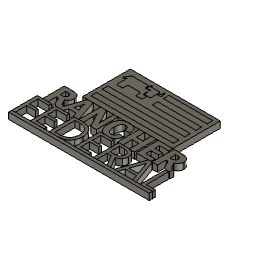
rancher-federal-stand (Autodesk Fusion 360 design; units mm, degrees)
Autodesk Fusion 360 part; units mm, degrees
sketch "Sketch1" plane through (0, 0, 0) normal (0, 0, 1) x (1, 0, 0)
  line L0 (14.2062, -89.6558) -> (3.2469, -89.6558)
  line L1 (3.2469, -89.6558) -> (-8.7202, -125.3052)
  spline S0 degree 3 poles (-8.7202, -125.3052) (-9.2241, -125.4312) (-9.791, -125.5571) (-10.2948, -125.5571) knots 0 0 0 0 1 1 1 1
  spline S1 degree 3 poles (-10.2948, -125.5571) (-14.1369, -125.5571) (-15.3336, -121.4631) (-17.1602, -117.81) knots 0 0 0 0 1 1 1 1
  spline S2 degree 3 poles (-17.1602, -117.81) (-17.853, -116.2354) (-18.9237, -114.7867) (-20.1834, -113.653) knots 0 0 0 0 1 1 1 1
  spline S3 degree 3 poles (-20.1834, -113.653) (-15.8375, -112.2673) (-11.3656, -108.3623) (-11.3656, -101.8119) knots 0 0 0 0 1 1 1 1
  spline S4 degree 3 poles (-11.3656, -101.8119) (-11.3656, -93.8128) (-17.0972, -89.6558) (-25.6631, -89.6558) knots 0 0 0 0 1 1 1 1
  line L2 (-25.6631, -89.6558) -> (-43.6138, -89.6558)
  line L3 (-43.6138, -89.6558) -> (-43.6138, -133.3683)
  line L4 (-43.6138, -133.3683) -> (-32.7804, -133.3683)
  line L5 (-32.7804, -133.3683) -> (-32.7804, -115.9834)
  line L6 (-32.7804, -115.9834) -> (-30.324, -115.9834)
  spline S5 degree 3 poles (-30.324, -115.9834) (-27.9306, -115.9834) (-26.104, -121.4631) (-24.8443, -124.5494) knots 0 0 0 0 1 1 1 1
  spline S6 degree 3 poles (-24.8443, -124.5494) (-21.821, -131.4777) (-18.8607, -133.4932) (-13.696, -133.4932) knots 0 0 0 0 1 1 1 1
  spline S7 degree 3 poles (-13.696, -133.4932) (-12.9402, -133.4302) (-12.1844, -133.3672) (-11.4285, -133.3042) knots 0 0 0 0 1 1 1 1
  line L7 (-11.4285, -133.3042) -> (-1.9808, -133.3042)
  line L8 (-1.9808, -133.3042) -> (0.6645, -124.9903)
  line L9 (0.6645, -124.9903) -> (15.277, -124.9903)
  line L10 (15.277, -124.9903) -> (18.0267, -133.4312)
  line L11 (18.0267, -133.4312) -> (28.9876, -133.4312)
  line L12 (28.9876, -133.4312) -> (14.2062, -89.6558)
  line L13 (-28.9383, -108.2363) -> (-32.8434, -108.2363)
  line L14 (-32.8434, -108.2363) -> (-32.8434, -97.5289)
  line L15 (-32.8434, -97.5289) -> (-27.6157, -97.5289)
  spline S8 degree 3 poles (-27.6157, -97.5289) (-24.6554, -97.5289) (-22.199, -98.7886) (-22.199, -102.6307) knots 0 0 0 0 1 1 1 1
  spline S9 degree 3 poles (-22.199, -102.6307) (-22.199, -107.2915) (-25.8521, -108.2363) (-28.9383, -108.2363) knots 0 0 0 0 1 1 1 1
  line L16 (3.2469, -117.0542) -> (6.2701, -107.7954)
  spline S10 degree 3 poles (6.2701, -107.7954) (7.026, -105.339) (7.5298, -102.8826) (7.9078, -100.3632) knots 0 0 0 0 1 1 1 1
  line L17 (7.9078, -100.3632) -> (8.1597, -100.3632)
  spline S11 degree 3 poles (8.1597, -100.3632) (8.4746, -102.8826) (8.9785, -105.402) (9.6713, -107.8584) knots 0 0 0 0 1 1 1 1
  line L18 (9.6713, -107.8584) -> (12.6316, -117.0542)
  line L19 (12.6316, -117.0542) -> (3.2469, -117.0542)
  line L20 (29.3856, -89.6558) -> (40.9747, -89.6558)
  line L21 (40.9747, -89.6558) -> (52.438, -111.3226)
  spline S12 degree 3 poles (52.438, -111.3226) (53.3828, -113.2121) (54.7054, -116.4873) (55.7132, -119.0697) knots 0 0 0 0 1 1 1 1
  line L22 (55.7132, -119.0697) -> (55.9651, -119.0697)
  spline S13 degree 3 poles (55.9651, -119.0697) (55.8392, -116.6133) (55.5242, -113.0861) (55.5242, -110.5668) knots 0 0 0 0 1 1 1 1
  line L23 (55.5242, -110.5668) -> (55.5242, -89.6558)
  line L24 (55.5242, -89.6558) -> (64.4051, -89.6558)
  line L25 (64.4051, -89.6558) -> (64.4051, -133.3043)
  line L26 (64.4051, -133.3043) -> (53.0678, -133.3043)
  line L27 (53.0678, -133.3043) -> (41.1637, -111.7005)
  spline S14 degree 3 poles (41.1637, -111.7005) (39.967, -109.37) (38.8963, -107.0396) (38.0145, -104.5832) knots 0 0 0 0 1 1 1 1
  line L28 (38.0145, -104.5832) -> (37.7625, -104.5832)
  spline S15 degree 3 poles (37.7625, -104.5832) (37.9515, -107.0396) (38.2664, -109.9369) (38.2664, -112.3303) knots 0 0 0 0 1 1 1 1
  line L29 (38.2664, -112.3303) -> (38.2664, -133.4313)
  line L30 (38.2664, -133.4313) -> (29.3226, -133.4313)
  line L31 (29.3226, -133.4313) -> (29.3226, -89.6558)
  line L32 (29.3226, -89.6558) -> (29.3856, -89.6558)
  spline S16 degree 3 poles (66.6725, -111.1966) (66.6725, -95.3874) (74.4826, -88.9) (86.5757, -88.9) knots 0 0 0 0 1 1 1 1
  spline S17 degree 3 poles (86.5757, -88.9) (99.2986, -88.9) (104.4634, -95.8913) (103.0147, -105.339) knots 0 0 0 0 1 1 1 1
  line L33 (103.0147, -105.339) -> (92.9372, -106.2208)
  spline S18 degree 3 poles (92.9372, -106.2208) (94.0709, -99.2925) (91.2996, -96.5212) (86.3868, -96.5212) knots 0 0 0 0 1 1 1 1
  spline S19 degree 3 poles (86.3868, -96.5212) (81.6629, -96.5212) (77.8208, -100.0483) (77.8208, -111.2596) knots 0 0 0 0 1 1 1 1
  spline S20 degree 3 poles (77.8208, -111.2596) (77.8208, -123.1637) (81.9778, -126.187) (86.7017, -126.187) knots 0 0 0 0 1 1 1 1
  spline S21 degree 3 poles (86.7017, -126.187) (91.1736, -126.187) (94.7637, -123.4156) (94.0079, -117.684) knots 0 0 0 0 1 1 1 1
  line L34 (94.0079, -117.684) -> (103.4556, -118.6288)
  spline S22 degree 3 poles (103.4556, -118.6288) (104.1484, -127.5097) (97.787, -133.9971) (86.1348, -133.9971) knots 0 0 0 0 1 1 1 1
  spline S23 degree 3 poles (86.1348, -133.9971) (74.3567, -134.1231) (66.7355, -127.1317) (66.6725, -111.1966) knots 0 0 0 0 1 1 1 1
  line L35 (106.9828, -89.6558) -> (117.7532, -89.6558)
  line L36 (117.7532, -89.6558) -> (117.7532, -106.1578)
  line L37 (117.7532, -106.1578) -> (131.0429, -106.1578)
  line L38 (131.0429, -106.1578) -> (131.0429, -89.6558)
  line L39 (131.0429, -89.6558) -> (141.8133, -89.6558)
  line L40 (141.8133, -89.6558) -> (141.8133, -134.1292)
  line L41 (141.8133, -134.1292) -> (131.0429, -134.1292)
  line L42 (131.0429, -134.1292) -> (131.0429, -114.8497)
  line L43 (131.0429, -114.8497) -> (117.7532, -114.8497)
  line L44 (117.7532, -114.8497) -> (117.7532, -133.3672)
  line L45 (117.7532, -133.3672) -> (106.9828, -133.3672)
  line L46 (106.9828, -133.3672) -> (106.9828, -89.6558)
  line L47 (144.8996, -89.6558) -> (173.8096, -89.6558)
  line L48 (173.8096, -89.6558) -> (173.8096, -97.7179)
  line L49 (173.8096, -97.7179) -> (155.733, -97.7179)
  line L50 (155.733, -97.7179) -> (155.733, -107.1026)
  line L51 (155.733, -107.1026) -> (170.9123, -107.1026)
  line L52 (170.9123, -107.1026) -> (170.9123, -115.1017)
  line L53 (170.9123, -115.1017) -> (155.733, -115.1017)
  line L54 (155.733, -115.1017) -> (155.733, -125.3052)
  line L55 (155.733, -125.3052) -> (174.4394, -125.3052)
  line L56 (174.4394, -125.3052) -> (174.4394, -133.6974)
  line L57 (174.4394, -133.6974) -> (144.8996, -133.6974)
  line L58 (144.8996, -133.6974) -> (144.8996, -89.6558)
  line L59 (176.5179, -89.6558) -> (194.4686, -89.6558)
  spline S24 degree 3 poles (194.4686, -89.6558) (203.0345, -89.6558) (208.7662, -93.8128) (208.7662, -101.8119) knots 0 0 0 0 1 1 1 1
  spline S25 degree 3 poles (208.7662, -101.8119) (208.7662, -108.3623) (204.2942, -112.2673) (199.9483, -113.653) knots 0 0 0 0 1 1 1 1
  spline S26 degree 3 poles (199.9483, -113.653) (201.208, -114.7867) (202.2787, -116.2354) (202.9715, -117.81) knots 0 0 0 0 1 1 1 1
  spline S27 degree 3 poles (202.9715, -117.81) (204.7981, -121.4631) (205.9948, -125.5571) (209.8369, -125.5571) knots 0 0 0 0 1 1 1 1
  spline S28 degree 3 poles (209.8369, -125.5571) (210.4038, -125.5571) (211.0336, -125.4312) (211.6005, -125.2422) knots 0 0 0 0 1 1 1 1
  line L60 (211.6005, -125.2422) -> (210.7817, -132.9263)
  spline S29 degree 3 poles (210.7817, -132.9263) (209.333, -133.2413) (207.8844, -133.4302) (206.4357, -133.4932) knots 0 0 0 0 1 1 1 1
  spline S30 degree 3 poles (206.4357, -133.4932) (201.2709, -133.4932) (198.3107, -131.4777) (195.2244, -124.5494) knots 0 0 0 0 1 1 1 1
  spline S31 degree 3 poles (195.2244, -124.5494) (193.9647, -121.4631) (192.1382, -115.9834) (189.7447, -115.9834) knots 0 0 0 0 1 1 1 1
  line L61 (189.7447, -115.9834) -> (187.2883, -115.9834)
  line L62 (187.2883, -115.9834) -> (187.2883, -133.7493)
  line L63 (187.2883, -133.7493) -> (176.5179, -133.7493)
  line L64 (176.5179, -133.7493) -> (176.5179, -89.6558)
  line L65 (187.3513, -97.5289) -> (187.3513, -108.2363)
  line L66 (187.3513, -108.2363) -> (191.2564, -108.2363)
  spline S32 degree 3 poles (191.2564, -108.2363) (194.3427, -108.2363) (197.9958, -107.2915) (197.9958, -102.6307) knots 0 0 0 0 1 1 1 1
  spline S33 degree 3 poles (197.9958, -102.6307) (197.9958, -98.7886) (195.5394, -97.5289) (192.5791, -97.5289) knots 0 0 0 0 1 1 1 1
  line L67 (192.5791, -97.5289) -> (187.3513, -97.5289)
  line L68 (77.6602, -0.8188) -> (165.5239, -0.8188)
  line L69 (165.5239, -0.8188) -> (165.5239, -12.0931)
  line L70 (165.5239, -12.0931) -> (77.6602, -12.0931)
  line L71 (77.6602, -12.0931) -> (77.6602, -0.8188)
  line L72 (77.6602, -23.3673) -> (165.5239, -23.3673)
  line L73 (165.5239, -23.3673) -> (165.5239, -34.6416)
  line L74 (165.5239, -34.6416) -> (77.6602, -34.6416)
  line L75 (77.6602, -34.6416) -> (77.6602, -23.3673)
  line L76 (0, -45.9159) -> (165.5239, -45.9159)
  line L77 (165.5239, -45.9159) -> (165.5239, -57.1902)
  line L78 (165.5239, -57.1902) -> (0, -57.1902)
  line L79 (0, -57.1902) -> (0, -45.9159)
  line L80 (0, -68.5274) -> (165.5239, -68.5274)
  line L81 (165.5239, -68.5274) -> (165.5239, -79.8017)
  line L82 (165.5239, -79.8017) -> (0, -79.8017)
  line L83 (0, -79.8017) -> (0, -68.5274)
  line L84 (72.0546, -8.251) -> (71.2987, -3.5901)
  spline S34 degree 3 poles (71.2987, -3.5901) (71.0468, -2.0785) (70.4799, -0.8188) (69.9761, -0.8188) knots 0 0 0 0 1 1 1 1
  spline S35 degree 3 poles (69.9761, -0.8188) (69.4722, -0.8188) (69.1573, -2.0785) (69.1573, -3.5901) knots 0 0 0 0 1 1 1 1
  line L85 (69.1573, -3.5901) -> (69.1573, -4.8498)
  spline S36 degree 3 poles (69.1573, -4.8498) (69.1573, -6.3615) (67.8976, -7.5582) (66.3859, -7.5582) knots 0 0 0 0 1 1 1 1
  line L86 (66.3859, -7.5582) -> (64.8743, -7.5582)
  line L87 (64.8743, -7.5582) -> (64.8743, -10.9593)
  line L88 (64.8743, -10.9593) -> (69.7871, -10.9593)
  spline S37 degree 3 poles (69.7871, -10.9593) (71.0468, -11.0223) (72.1175, -10.0146) (72.1805, -8.7549) knots 0 0 0 0 1 1 1 1
  spline S38 degree 3 poles (72.1805, -8.7549) (72.1175, -8.5659) (72.1175, -8.377) (72.0546, -8.251) knots 0 0 0 0 1 1 1 1
  line L89 (61.0322, -4.283) -> (45.6639, -4.283)
  spline S39 degree 3 poles (45.6639, -4.283) (45.601, -4.283) (45.475, -4.283) (45.412, -4.283) knots 0 0 0 0 1 1 1 1
  line L90 (45.412, -4.283) -> (45.412, -3.5271)
  spline S40 degree 3 poles (45.412, -3.5271) (45.412, -2.0155) (45.0341, -0.7558) (44.5932, -0.7558) knots 0 0 0 0 1 1 1 1
  spline S41 degree 3 poles (44.5932, -0.7558) (44.1523, -0.7558) (43.5225, -2.0155) (43.2705, -3.4642) knots 0 0 0 0 1 1 1 1
  line L91 (43.2705, -3.4642) -> (42.4517, -8.188)
  spline S42 degree 3 poles (42.4517, -8.188) (42.1998, -9.4477) (42.9556, -10.6444) (44.2153, -10.8964) knots 0 0 0 0 1 1 1 1
  spline S43 degree 3 poles (44.2153, -10.8964) (44.4043, -10.9593) (44.5932, -10.9593) (44.7822, -10.9593) knots 0 0 0 0 1 1 1 1
  line L92 (44.7822, -10.9593) -> (49.3801, -10.9593)
  spline S44 degree 3 poles (49.3801, -10.9593) (49.8209, -10.9593) (50.2618, -10.8964) (50.7027, -10.7074) knots 0 0 0 0 1 1 1 1
  spline S45 degree 3 poles (50.7027, -10.7074) (50.5768, -11.5262) (49.8839, -12.0931) (49.0651, -12.0931) knots 0 0 0 0 1 1 1 1
  line L93 (49.0651, -12.0931) -> (42.5777, -12.0931)
  spline S46 degree 3 poles (42.5777, -12.0931) (41.6329, -12.0931) (40.8771, -11.3373) (40.8771, -10.3925) knots 0 0 0 0 1 1 1 1
  spline S47 degree 3 poles (40.8771, -10.3925) (40.8771, -10.3295) (40.8771, -10.2035) (40.8771, -10.1405) knots 0 0 0 0 1 1 1 1
  line L94 (40.8771, -10.1405) -> (41.507, -6.2355)
  spline S48 degree 3 poles (41.507, -6.2355) (41.6329, -5.2907) (41.0661, -4.4719) (40.1213, -4.283) knots 0 0 0 0 1 1 1 1
  spline S49 degree 3 poles (40.1213, -4.283) (40.0583, -4.283) (39.9323, -4.283) (39.8693, -4.283) knots 0 0 0 0 1 1 1 1
  line L95 (39.8693, -4.283) -> (7.6841, -4.283)
  spline S50 degree 3 poles (7.6841, -4.283) (6.9913, -4.283) (6.4244, -4.6609) (6.1725, -5.2907) knots 0 0 0 0 1 1 1 1
  line L96 (6.1725, -5.2907) -> (0.063, -14.4865)
  spline S51 degree 3 poles (0.063, -14.4865) (-0.063, -14.6125) (0, -14.8644) (0.063, -14.9904) knots 0 0 0 0 1 1 1 1
  line L97 (0.063, -14.9904) -> (1.2597, -16.376)
  spline S52 degree 3 poles (1.2597, -16.376) (1.3857, -16.565) (1.6376, -16.565) (1.8266, -16.439) knots 0 0 0 0 1 1 1 1
  line L98 (1.8266, -16.439) -> (5.9206, -13.2268)
  line L99 (5.9206, -13.2268) -> (5.9206, -32.941)
  spline S53 degree 3 poles (5.9206, -32.941) (5.9206, -33.8858) (6.6764, -34.6416) (7.5582, -34.6416) knots 0 0 0 0 1 1 1 1
  line L100 (7.558, -34.6416) -> (16.7539, -34.6416)
  spline S54 degree 3 poles (16.7539, -34.6416) (17.6987, -34.6416) (18.4545, -33.8858) (18.4545, -32.941) knots 0 0 0 0 1 1 1 1
  line L101 (18.4545, -32.941) -> (18.4545, -26.0757)
  spline S55 degree 3 poles (18.4545, -26.0757) (18.4545, -25.1309) (19.2104, -24.3751) (20.1551, -24.3751) knots 0 0 0 0 1 1 1 1
  line L102 (20.1551, -24.3751) -> (42.9556, -24.3751)
  spline S56 degree 3 poles (42.9556, -24.3751) (43.9004, -24.3751) (44.6562, -25.1309) (44.6562, -26.0757) knots 0 0 0 0 1 1 1 1
  line L103 (44.6562, -26.0757) -> (44.6562, -32.941)
  spline S57 degree 3 poles (44.6562, -32.941) (44.6562, -33.8858) (45.412, -34.6416) (46.2938, -34.6416) knots 0 0 0 0 1 1 1 1
  line L104 (46.2938, -34.6416) -> (55.4896, -34.6416)
  spline S58 degree 3 poles (55.4896, -34.6416) (56.4343, -34.6416) (57.1901, -33.8858) (57.1901, -32.941) knots 0 0 0 0 1 1 1 1
  line L105 (57.1901, -32.941) -> (57.1901, -25.5088)
  line L106 (57.1901, -25.5088) -> (52.3403, -25.5088)
  spline S59 degree 3 poles (52.3403, -25.5088) (50.8287, -25.5088) (49.569, -24.2491) (49.569, -22.7375) knots 0 0 0 0 1 1 1 1
  line L107 (49.569, -22.7375) -> (49.569, -18.0136)
  spline S60 degree 3 poles (49.569, -18.0136) (49.569, -17.1319) (50.0099, -16.313) (50.7027, -15.8092) knots 0 0 0 0 1 1 1 1
  line L108 (50.7027, -15.8092) -> (50.7027, -21.4778)
  spline S61 degree 3 poles (50.7027, -21.4778) (50.7027, -22.9894) (51.9624, -24.2491) (53.4741, -24.2491) knots 0 0 0 0 1 1 1 1
  line L109 (53.4741, -24.2491) -> (60.9063, -24.2491)
  spline S62 degree 3 poles (60.9063, -24.2491) (62.4179, -24.2491) (63.6776, -22.9894) (63.6776, -21.4778) knots 0 0 0 0 1 1 1 1
  line L110 (63.6776, -21.4778) -> (63.6776, -6.9913)
  spline S63 degree 3 poles (63.6776, -6.9913) (63.7406, -5.4797) (62.5439, -4.283) (61.0322, -4.283) knots 0 0 0 0 1 1 1 1
  line L111 (-6.9304, 6.1202) -> (173.8096, 6.1202)
  line L112 (173.8096, 6.1202) -> (173.8096, -89.6558)
  line L113 (173.8096, -89.6558) -> (-6.9304, -89.6558)
  line L114 (-6.9304, -89.6558) -> (-6.9304, 6.1202)
  line L115 (-25.4398, -133.357) -> (-25.4398, -138.7816)
  line L116 (-25.4398, -138.7816) -> (-47.6511, -138.7816)
  line L117 (-47.6511, -138.7816) -> (-47.6511, -156.0081)
  line L118 (-47.6511, -156.0081) -> (-29.6182, -156.0081)
  line L119 (-29.6182, -156.0081) -> (-29.6182, -161.4326)
  line L120 (-29.6182, -161.4326) -> (-47.6511, -161.4326)
  line L121 (-47.6511, -161.4326) -> (-47.6511, -184.4502)
  line L122 (-47.6511, -184.4502) -> (-54.3218, -184.4502)
  line L123 (-54.3218, -184.4502) -> (-54.3218, -133.357)
  line L124 (-54.3218, -133.357) -> (-25.4398, -133.357)
  line L125 (-10.7056, -138.7816) -> (-10.7056, -155.8615)
  line L126 (-10.7056, -155.8615) -> (7.9137, -155.8615)
  line L127 (7.9137, -155.8615) -> (7.9137, -161.3593)
  line L128 (7.9137, -161.3593) -> (-10.7056, -161.3593)
  line L129 (-10.7056, -161.3593) -> (-10.7056, -178.9524)
  line L130 (-10.7056, -178.9524) -> (10.1128, -178.9524)
  line L131 (10.1128, -178.9524) -> (10.1128, -184.4502)
  line L132 (10.1128, -184.4502) -> (-17.3763, -184.4502)
  line L133 (-17.3763, -184.4502) -> (-17.3763, -133.2837)
  line L134 (-17.3763, -133.2837) -> (10.1128, -133.2837)
  line L135 (10.1128, -133.2837) -> (10.1128, -138.7816)
  line L136 (10.1128, -138.7816) -> (-10.7056, -138.7816)
  spline S64 degree 2 poles (36.1359, -133.357) (44.4926, -133.357) (50.5769, -136.5091) knots 0 0 0 1 1 1
  spline S65 degree 2 poles (50.5769, -136.5091) (56.7345, -139.5879) (59.9599, -145.379) knots 0 0 0 1 1 1
  spline S66 degree 2 poles (59.9599, -145.379) (63.2586, -151.17) (63.2586, -159.0136) knots 0 0 0 1 1 1
  spline S67 degree 2 poles (63.2586, -159.0136) (63.2586, -166.8572) (59.9599, -172.6482) knots 0 0 0 1 1 1
  spline S68 degree 2 poles (59.9599, -172.6482) (56.7345, -178.366) (50.5769, -181.4448) knots 0 0 0 1 1 1
  spline S69 degree 2 poles (50.5769, -181.4448) (44.4926, -184.4502) (36.1359, -184.4502) knots 0 0 0 1 1 1
  line L137 (36.1359, -184.4502) -> (20.2289, -184.4502)
  line L138 (20.2289, -184.4502) -> (20.2289, -133.357)
  line L139 (20.2289, -133.357) -> (36.1359, -133.357)
  spline S70 degree 2 poles (36.1359, -178.9524) (46.032, -178.9524) (51.2367, -173.7478) knots 0 0 0 1 1 1
  spline S71 degree 2 poles (51.2367, -173.7478) (56.4413, -168.4699) (56.4413, -159.0136) knots 0 0 0 1 1 1
  spline S72 degree 2 poles (56.4413, -159.0136) (56.4413, -149.484) (51.1634, -144.1328) knots 0 0 0 1 1 1
  spline S73 degree 2 poles (51.1634, -144.1328) (45.9587, -138.7816) (36.1359, -138.7816) knots 0 0 0 1 1 1
  line L140 (36.1359, -138.7816) -> (26.8996, -138.7816)
  line L141 (26.8996, -138.7816) -> (26.8996, -178.9524)
  line L142 (26.8996, -178.9524) -> (36.1359, -178.9524)
  line L143 (78.7258, -138.7816) -> (78.7258, -155.8615)
  line L144 (78.7258, -155.8615) -> (97.3452, -155.8615)
  line L145 (97.3452, -155.8615) -> (97.3452, -161.3593)
  line L146 (97.3452, -161.3593) -> (78.7258, -161.3593)
  line L147 (78.7258, -161.3593) -> (78.7258, -178.9524)
  line L148 (78.7258, -178.9524) -> (99.5443, -178.9524)
  line L149 (99.5443, -178.9524) -> (99.5443, -184.4502)
  line L150 (99.5443, -184.4502) -> (72.0551, -184.4502)
  line L151 (72.0551, -184.4502) -> (72.0551, -133.2837)
  line L152 (72.0551, -133.2837) -> (99.5443, -133.2837)
  line L153 (99.5443, -133.2837) -> (99.5443, -138.7816)
  line L154 (99.5443, -138.7816) -> (78.7258, -138.7816)
  line L155 (136.5631, -184.4502) -> (124.3945, -163.5585)
  line L156 (124.3945, -163.5585) -> (116.331, -163.5585)
  line L157 (116.331, -163.5585) -> (116.331, -184.4502)
  line L158 (116.331, -184.4502) -> (109.6603, -184.4502)
  line L159 (109.6603, -184.4502) -> (109.6603, -133.357)
  line L160 (109.6603, -133.357) -> (126.1538, -133.357)
  spline S74 degree 2 poles (126.1538, -133.357) (131.9449, -133.357) (135.9033, -135.3363) knots 0 0 0 1 1 1
  spline S75 degree 2 poles (135.9033, -135.3363) (139.9351, -137.3155) (141.9143, -140.6875) knots 0 0 0 1 1 1
  spline S76 degree 2 poles (141.9143, -140.6875) (143.8935, -144.0595) (143.8935, -148.3844) knots 0 0 0 1 1 1
  spline S77 degree 2 poles (143.8935, -148.3844) (143.8935, -153.6624) (140.8147, -157.6941) knots 0 0 0 1 1 1
  spline S78 degree 2 poles (140.8147, -157.6941) (137.8092, -161.7259) (131.725, -163.0453) knots 0 0 0 1 1 1
  line L161 (131.725, -163.0453) -> (144.5532, -184.4502)
  line L162 (144.5532, -184.4502) -> (136.5631, -184.4502)
  line L163 (116.331, -158.2072) -> (126.1538, -158.2072)
  spline S79 degree 2 poles (126.1538, -158.2072) (131.5784, -158.2072) (134.2906, -155.5683) knots 0 0 0 1 1 1
  spline S80 degree 2 poles (134.2906, -155.5683) (137.0029, -152.856) (137.0029, -148.3844) knots 0 0 0 1 1 1
  spline S81 degree 2 poles (137.0029, -148.3844) (137.0029, -143.8396) (134.2906, -141.3472) knots 0 0 0 1 1 1
  spline S82 degree 2 poles (134.2906, -141.3472) (131.6517, -138.8549) (126.1538, -138.8549) knots 0 0 0 1 1 1
  line L164 (126.1538, -138.8549) -> (116.331, -138.8549)
  line L165 (116.331, -138.8549) -> (116.331, -158.2072)
  line L166 (184.4309, -173.0881) -> (162.1463, -173.0881)
  line L167 (162.1463, -173.0881) -> (158.0413, -184.4502)
  line L168 (158.0413, -184.4502) -> (151.004, -184.4502)
  line L169 (151.004, -184.4502) -> (169.4768, -133.6503)
  line L170 (169.4768, -133.6503) -> (177.1737, -133.6503)
  line L171 (177.1737, -133.6503) -> (195.5731, -184.4502)
  line L172 (195.5731, -184.4502) -> (188.5359, -184.4502)
  line L173 (188.5359, -184.4502) -> (184.4309, -173.0881)
  line L174 (182.525, -167.6635) -> (173.2886, -141.8604)
  line L175 (173.2886, -141.8604) -> (164.0522, -167.6635)
  line L176 (164.0522, -167.6635) -> (182.525, -167.6635)
  line L177 (210.3074, -179.0257) -> (228.1936, -179.0257)
  line L178 (228.1936, -179.0257) -> (228.1936, -184.4502)
  line L179 (228.1936, -184.4502) -> (203.6366, -184.4502)
  line L180 (203.6366, -184.4502) -> (203.6366, -133.357)
  line L181 (203.6366, -133.357) -> (210.3074, -133.357)
  line L182 (210.3074, -133.357) -> (210.3074, -179.0257)
  line L183 (-54.3218, -184.4502) -> (228.1936, -184.4502)
  line L184 (228.1936, -184.4502) -> (228.1936, -190.9812)
  line L185 (228.1936, -190.9812) -> (-54.3218, -190.9812)
  line L186 (-54.3218, -190.9812) -> (-54.3218, -184.4502)
  constraint horizontal L111
  constraint vertical L112
  constraint horizontal L113
  constraint vertical L114
  constraint horizontal L104
  constraint horizontal L183
  constraint vertical L184
  constraint horizontal L185
  constraint vertical L186
sketch "Sketch2" plane through (0, 0, 0) normal (0, 0, 1) x (1, 0, 0)
extrude "Extrude8" add sketch "Sketch1" along normal blind 12.7 contours L0 L20 L24 L32 S16 S17 L35 L39 L47 L111 L112 L113 L114 makes body 1
extrude "Extrude9" add sketch "Sketch1" along normal blind 12.7 separate body contours L11 L12 L29 L30 L31 S64 S65 S66 S67 S68 S69 L137 L138 L139 L183 | L11 L12 L138 L139 | L29 L30 L31 S64 L139 | S6 S7 L7 L8 L125 L126 L127 L128 L129 L130 L131 L132 L133 L134 L135 L136 L183 | S22 S23 L143 L144 L145 L146 L147 L148 L149 L150 L151 L152 L153 L154 L183 | S6 S7 L7 L8 L134 | L3 L4 L5 L115 L116 L117 L118 L119 L120 L121 L122 L123 L124 L183 | L56 L57 L169 L170 | L56 L57 L63 L64 L166 L167 L168 L169 L170 L171 L172 L173 L183 | L41 L42 L44 L45 L155 L156 L157 L158 L159 L160 S74 S75 S76 S77 S78 L161 L162 L183 | S22 S23 L152 | L3 L4 L5 L124 | L41 L42 S74 | L63 L64 L170 L171 | S29 S30 L177 L178 L179 L180 L181 L182 L183 | S29 S30 L181 | L68 L69 L70 L71 | L72 L73 L74 L75 | L76 L77 L78 L79 | L80 L81 L82 L83 makes body 2 at (111.8839, -158.6749, 0) makes body 3 at (-54.3218, -167.4192, 4.2333) makes body 4 at (136.236, -0.8188, 8.4667) makes body 5 at (55.1746, -68.5274, 4.2333) makes body 6 at (74.2787, -159.6978, 0) makes body 7 at (185.0906, -161.9213, 0) makes body 8 at (-15.1528, -159.6978, 0) makes body 9 at (136.236, -23.3673, 8.4667) makes body 10 at (55.1746, -45.9159, 4.2333) makes body 11 at (22.4524, -165.5866, 0) makes body 12 at (203.6366, -167.4192, 4.2333)
extrude "Extrude10" add sketch "Sketch1" along normal blind 12.7 separate body contours L0 L1 S0 S1 S2 S3 S4 L2 L3 L5 L6 S5 S6 L8 L9 L10 L11 L12 L113 L124 L134 L138 L139 | L20 L21 S12 L22 S13 L23 L24 L25 L26 L27 S14 L28 S15 L29 L31 L32 L113 S64 L139 | L47 L48 L49 L50 L51 L52 L53 L54 L55 L56 L57 L58 L113 L169 L170 | S16 S17 L33 S18 S19 S20 S21 L34 S22 S23 L113 L152 | L35 L36 L37 L38 L39 L40 L41 L42 L43 L44 L45 L46 L113 L159 L160 S74 | L59 S24 S25 S26 S27 S28 L60 S29 S30 S31 L61 L62 L63 L64 L170 L171 L181 | L84 S34 S35 L85 S36 L86 L87 L88 S37 S38 | L89 S39 L90 S40 S41 L91 S42 S43 L92 S44 S45 L93 S46 S47 L94 S48 S49 L95 S50 L96 S51 L97 S52 L98 L99 S53 L100 S54 L101 S55 L102 S56 L103 S57 L104 S58 L105 L106 S59 L107 S60 L108 S61 L109 S62 L110 S63 makes body 13 at (-40.0236, -110.4164, 0) makes body 14 at (148.5107, -112.8183, 0) makes body 15 at (138.2232, -112.8783, 0) makes body 16 at (22.5695, -10.9803, 0) makes body 17 at (32.3039, -111.7811, 0) makes body 18 at (180.1291, -110.5141, 0) makes body 19 at (86.1044, -130.912, 0) makes body 20 at (68.1495, -10.9593, 8.4667)
extrude "Extrude11" add sketch "Sketch1" along normal blind 12.7 separate body contours L122 L132 L137 L150 L158 L162 L168 L172 L179 L183 L184 L185 L186 makes body 21
extrude "Extrude2" [suppressed]
